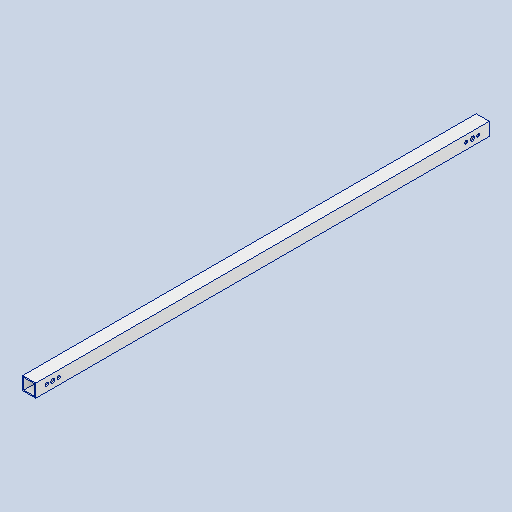
# Autodesk Inventor part: roller-hand-v2-ASP-1
Saved by Autodesk Inventor 2025.1 (Build 291241000, 241)
## iProperties
Created: 2024-10-06
Part Number: roller-hand-v2-ASP-1
Material: アルミニウム 6061
Document SubType Name: Modeling
Designer: haruy
Density: 2.7 g/cm^3
Appearance: アルミニウム - フラット
Author: haruy
Autodesk Inventor part; units mm, degrees
ref_plane "YZ Plane" through (0, 0, 0) normal (1, 0, 0) x (0, 1, 0)
ref_plane "XZ Plane" through (0, 0, 0) normal (0, 1, 0) x (-1, 0, 0)
ref_plane "XY Plane" through (0, 0, 0) normal (0, 0, 1) x (1, 0, 0)
derived "roller-hand-v2-Sketch-Base.ipt"
sketch "スケッチ2" plane through (0, 200, 0) normal (0, 1, 0) x (-1, 0, 0)
  line L0 (0, 0) -> (280, 0)
  line L1 (280, 0) -> (280, -18)
  line L2 (280, -18) -> (0, -18)
  line L3 (0, -18) -> (0, 0)
  line L4 (-5, 116.1253) -> (-8, 116.1253)
  line L5 (-8, 116.1253) -> (-8, -29.5691)
  line L6 (-8, -29.5691) -> (-5, -29.5691)
  line L7 (-5, -29.5691) -> (-5, 116.1253)
  line L8 (-5, 52.6222) -> (66.2, 52.6222)
  line L9 (66.2, 52.6222) -> (66.2, 20.6222)
  line L10 (66.2, 20.6222) -> (-5, 20.6222)
  line L11 (-5, 20.6222) -> (-5, 52.6222)
  line L12 (-5, 46.6222) -> (-9, 46.6222)
  line L13 (-9, 46.6222) -> (-9, 26.6222)
  line L14 (-9, 26.6222) -> (-5, 26.6222)
  line L15 (-5, 26.6222) -> (-5, 46.6222)
  line L16 (-9, 39.6222) -> (-23.8, 39.6222)
  line L17 (-23.8, 39.6222) -> (-23.8, 33.6222)
  line L18 (-23.8, 33.6222) -> (-9, 33.6222)
  line L19 (-9, 33.6222) -> (-9, 39.6222)
  line L20 (-14, 45.0445) -> (-20, 45.0445)
  line L21 (-20, 45.0445) -> (-20, 23.8894)
  line L22 (-20, 23.8894) -> (-14, 23.8894)
  line L23 (-14, 23.8894) -> (-14, 45.0445)
  line L24 (-20, 50.3109) -> (-26, 50.3109)
  line L25 (-26, 50.3109) -> (-26, 18.3109)
  line L26 (-26, 18.3109) -> (-20, 18.3109)
  line L27 (-20, 18.3109) -> (-20, 50.3109)
  line L28 (15, 0) -> (15, -18)
  line L29 (15, -4.3972) -> (-26, -4.3972)
  line L30 (-26, -4.3972) -> (-26, -16.3972)
  line L31 (-26, -16.3972) -> (15, -16.3972)
  line L32 (15, -16.3972) -> (15, -4.3972)
  line L33 (-14.8, 155.9564) -> (-17.8, 155.9564)
  line L34 (-17.8, 155.9564) -> (-17.8, 85.4399)
  line L35 (-17.8, 85.4399) -> (-14.8, 85.4399)
  line L36 (-14.8, 85.4399) -> (-14.8, 155.9564)
  line L37 (-21.6284, 147.0378) -> (100.6034, 147.0378)
  line L38 (100.6034, 147.0378) -> (100.6034, 143.0378)
  line L39 (100.6034, 143.0378) -> (-21.6284, 143.0378)
  line L40 (-21.6284, 143.0378) -> (-21.6284, 147.0378)
ref_plane "作業平面1" through (200, 0, 0) normal (1, 0, 0) x (0, 1, 0)
ref_plane "作業平面2" through (0, 200, 0) normal (0, 1, 0) x (-1, 0, 0)
sketch "スケッチ1" plane through (200, 0, 0) normal (1, 0, 0) x (0, 1, 0)
  circle A0 centre (0, 0) radius 4 projected
  circle A1 centre (15.5291, -57.9555) radius 9 projected
  circle A2 centre (7.2469, -27.0459) radius 16 projected
  circle A3 centre (27.4423, -44.1692) radius 2 projected
  circle A4 centre (74.6196, 7.5445) radius 2 projected
  line L0 (74.6196, 7.5445) -> (0, 0) construction
  line L1 (74.6196, 7.5445) -> (27.4423, -44.1692) projected
  line L2 (0, 0) -> (27.4423, -44.1692) projected
  line L3 (0, 0) -> (15.5291, -57.9555) projected
  circle A5 centre (0, -184.4555) radius 117.5 projected
  line L4 (155.3866, 15.5445) -> (-185.0808, 15.5445) projected
  circle A6 centre (0, 0) radius 60 construction
  line L5 (0, 0) -> (28.2083, -52.9555) projected
  circle A7 centre (0, 0) radius 52 construction
  circle A8 centre (36.6749, -36.864) radius 4 construction
  line L6 (74.6196, 7.5445) -> (36.6749, -36.864) construction
  circle A9 centre (27.4423, -44.1692) radius 9 projected
  circle A10 centre (74.6196, 7.5445) radius 9 projected
  circle A11 centre (15.5291, -57.9555) radius 12.5 projected
  circle A12 centre (0, 0) radius 11 projected
  circle A13 centre (7.2469, -27.0459) radius 9 projected
  circle A14 centre (15.5291, -57.9555) radius 16 projected
  circle A15 centre (7.2469, -27.0459) radius 16 projected
  line L7 (20.4525, -18.0119) -> (34.8704, -39.0876) projected
  circle A16 centre (15.5291, -57.9555) radius 12.5 projected
  line L8 (26.3809, -64.1595) -> (35.2556, -48.636) projected
  line L9 (-7.6622, -32.8526) -> (3.8814, -62.492) projected
  circle A17 centre (0, 0) radius 11 projected
  line L10 (73.9533, 16.5198) -> (-0.8143, 10.9698) projected
  line L11 (1.398, -10.9108) -> (75.7634, -1.3826) projected
  line L12 (9.946, 4.6986) -> (21.7139, -20.2116) projected
  line L13 (-10.9628, -0.9039) -> (-8.699, -28.3607) projected
  line L14 (0, -184.4555) -> (117.5, -184.4555) projected
  line L15 (68.6196, 23.0445) -> (80.6196, 23.0445)
  line L16 (80.6196, 23.0445) -> (80.6196, -184.4555)
  line L17 (80.6196, -184.4555) -> (68.6196, -184.4555)
  line L18 (68.6196, -184.4555) -> (68.6196, 23.0445)
  circle A18 centre (74.6196, 7.5445) radius 5.5
  circle A19 centre (74.6196, 13.0445) radius 1.5
  line L19 (74.6196, 13.0445) -> (74.6196, 7.5445)
  line L20 (68.6196, -7.9555) -> (68.6196, 199.5445)
  circle A20 centre (74.6196, 2.0445) radius 1.5
  circle A21 centre (74.6196, -376.4555) radius 2
  line L21 (68.6196, -391.9555) -> (80.6196, -391.9555)
  line L22 (80.6196, -391.9555) -> (80.6196, -184.4555)
  line L23 (68.6196, -184.4555) -> (68.6196, -391.9555)
  circle A22 centre (74.6196, -381.9555) radius 1.5
  circle A23 centre (74.6196, -370.9555) radius 1.5
  point P0 (58.75, -184.4555)
  dimension "d3" = 11
  dimension "d1" = 12
  dimension "d2" = 6
  dimension "d4" = 3
  dimension "d7" = 360
  dimension "d9" = 10
  dimension "d10" = 0
  constraints: 18 end point, 5 centre point, 5 symmetric about line, 2 parallel, 1 coincident, 1 horizontal, 1 horizontal alignment, 1 midpoint, 1 perpendicular, 1 vertical, 1 vertical alignment, 16 other
  measures "d1" distance of L16.end L17.end
  measures "d2" distance from line of L18 L0.start
  measures "d4" diameter of A19
  measures "d9" distance from line of L15 L19.start
  measures "d10" distance from line of point (58.75, -184.456) L17
extrude "押し出し1" add sketch "スケッチ1" along normal blind 12 contours L18 A10 L11 | L11 A10 L16 A5 L18 | L18 L10 A10 L4 | L4 A10 L18 | L18 L15 L16 L4 A10 L10 | L18 A10 L4 L16 | A10 L4 | A5 L16 L14 L18 | L23 L14 L22 A5 | A5 L22 L21 L23 | L4 L16 A10 | A4 L1 L19 | A4 L19 A19 A18 A20 L1 | L19 L1 A4 | A4 L1 A18 A19 L19 | L19 A18 A19 | A19 A18 L19 | A19 A18 | A20 A18 | A18 A20 | A21 | A22 | A23
shell "シェル1" thickness 1 removed faces 2 at (204, 72.6196, -391.9555) at (204, 76.6196, 23.0445)
hole "穴1" at (200, 74.6196, -381.9555) at (200, 74.6196, -370.9555) at (200, 74.6196, 2.0445) at (200, 74.6196, 13.0445) direction (1, 0, 0) diameter 3 end through all
hole "穴2" at (200, 74.6196, 7.5445) at (200, 74.6196, -376.4555) direction (1, 0, 0) diameter 4 end through all
